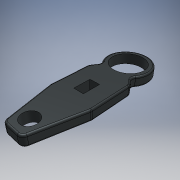
# Autodesk Inventor part: crossguard
Saved by Autodesk Inventor 2018 (Build 220112000, 112)
## iProperties
Created: 2020-12-01
Part Number: crossguard
Material: Všeobecné
Document SubType Name: Modeling
Designer: Jozko Mrkvicka
Density: 1 g/cm^3
Appearance: Výchozí
Author: Jozko Mrkvicka
Autodesk Inventor part; units mm, degrees
ref_plane "YZ Plane" through (0, 0, 0) normal (1, 0, 0) x (0, 1, 0)
ref_plane "XZ Plane" through (0, 0, 0) normal (0, 1, 0) x (-1, 0, 0)
ref_plane "XY Plane" through (0, 0, 0) normal (0, 0, 1) x (1, 0, 0)
sketch "Náčrt1" plane through (0, 0, 0) normal (0, 0, 1) x (1, 0, 0)
  line L0 (9.3423, 0) -> (16.6577, 0)
  line L1 (26, 28.3693) -> (26, 51.0917)
  line L2 (0, 51.0917) -> (0, 28.3693)
  circle A0 centre (13, 67) radius 10
  arc A1 (23.4879, 59.3186) -> (2.5121, 59.3186) centre (13, 67) ccw
  circle A2 centre (13, 8) radius 4.5
  line L3 (10, 43) -> (16, 43)
  line L4 (16, 43) -> (16, 33)
  line L5 (16, 33) -> (10, 33)
  line L6 (10, 33) -> (10, 43)
  line L7 (26, 51.0917) -> (26, 28.3693)
  line L8 (0, 28.3693) -> (0, 51.0917)
  line L9 (0.0896, 27.6417) -> (6.4319, 2.2724)
  line L10 (25.9104, 27.6417) -> (19.5681, 2.2724)
  line L11 (25.4962, 52.7558) -> (23.4121, 55.8819)
  line L12 (0.5038, 52.7558) -> (2.5879, 55.8819)
  arc A3 (6.4319, 2.2724) -> (9.3423, 0) centre (9.3423, 3) ccw
  arc A4 (16.6577, 0) -> (19.5681, 2.2724) centre (16.6577, 3) ccw
  arc A5 (0.5038, 52.7558) -> (0, 51.0917) centre (3, 51.0917) ccw
  arc A6 (26, 51.0917) -> (25.4962, 52.7558) centre (23, 51.0917) ccw
  arc A7 (23.4879, 59.3186) -> (23.4121, 55.8819) centre (25.9082, 57.546) ccw
  arc A8 (2.5879, 55.8819) -> (2.5121, 59.3186) centre (0.0918, 57.546) ccw
  arc A9 (25.9104, 27.6417) -> (26, 28.3693) centre (23, 28.3693) ccw
  arc A10 (0, 28.3693) -> (0.0896, 27.6417) centre (3, 28.3693) ccw
  point P0 (0, 0)
  point P1 (13, 38)
  point P2 (13, 38)
  point P3 (22.1538, 57.7692)
  point P4 (3.8462, 57.7692)
  dimension "d4" = 3
  dimension "d11" = 20
  constraints: 26 end point, 20 point on circle, 16 tangent, 11 centre point, 5 equal radius, 4 parallel, 2 horizontal, 2 perpendicular, 2 point on line, 1 coincident
  measures "d4" radius of A3
  measures "d11" diameter of A0
extrude "Vysunutí1" add sketch "Náčrt1" along normal blind 6
fillet "Zaoblení1" radius 1 16 edges at (25.8713, 51.961, 6) (24.4541, 54.3188, 6) (22.9089, 57.6122, 6) (13, 80, 6) (3.0911, 57.6122, 6) (1.5459, 54.3188, 6) (0.1287, 51.961, 6) (0, 39.7305, 6) (0.0225, 28.0028, 6) (3.2607, 14.9571, 6) (7.4961, 0.6354, 6) (13, 0, 6) (18.5039, 0.6354, 6) (22.7393, 14.9571, 6) (25.9775, 28.0028, 6) (26, 39.7305, 6)
fillet "Zaoblení2" radius 1 16 edges at (25.8713, 51.961, 0) (24.4541, 54.3188, 0) (22.9089, 57.6122, 0) (13, 80, 0) (3.0911, 57.6122, 0) (1.5459, 54.3188, 0) (0.1287, 51.961, 0) (0, 39.7305, 0) (0.0225, 28.0028, 0) (3.2607, 14.9571, 0) (7.4961, 0.6354, 0) (13, 0, 0) (18.5039, 0.6354, 0) (22.7393, 14.9571, 0) (25.9775, 28.0028, 0) (26, 39.7305, 0)
